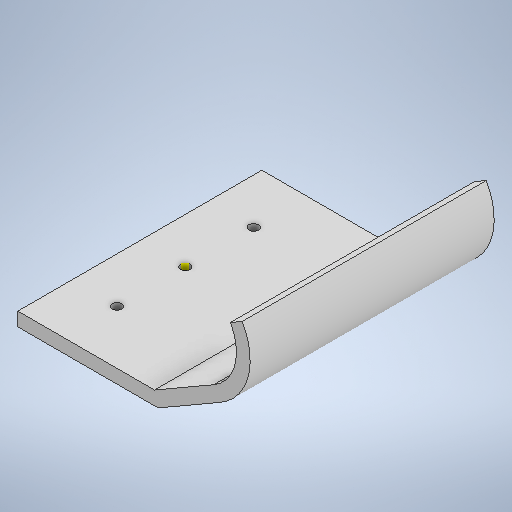
# Autodesk Inventor part: gripper_frame
Saved by Autodesk Inventor 2025.2 (Build 292293000, 293)
## iProperties
Created: 2025-08-01
Part Number: gripper_frame
Material: Generic
Document SubType Name: Modeling
Designer: LG
Density: 1 g/cm^3
Appearance: Default
Author: LG
Autodesk Inventor part; units mm, degrees
ref_plane "YZ Plane" through (0, 0, 0) normal (1, 0, 0) x (0, 1, 0)
ref_plane "XZ Plane" through (0, 0, 0) normal (0, 1, 0) x (-1, 0, 0)
ref_plane "XY Plane" through (0, 0, 0) normal (0, 0, 1) x (1, 0, 0)
sketch "Sketch1" plane through (0, 0, 0) normal (0, 1, 0) x (-1, 0, 0)
  line L0 (10, 26.78) -> (-20, 26.78)
  line L1 (-20, 26.78) -> (-20, -26.78)
  line L2 (-20, -26.78) -> (10, -26.78)
  line L3 (10, -26.78) -> (10, 26.78)
  point P0 (0, 0)
  dimension "d0" = 53.56
  dimension "d1" = 30
  dimension "d2" = 10
  dimension "d3" = 26.78
  constraints: 8 end point, 2 parallel, 1 horizontal, 1 perpendicular
  measures "d0" distance of L2.end L0.start
  measures "d1" distance of L1.end L2.end
  measures "d2" distance from line of point (0, 0) L3
  measures "d3" distance from line of L0 point (0, 0)
extrude "Extrusion1" add sketch "Sketch1" along normal blind 3
sketch "Sketch2" plane through (0, 3, 0) normal (0, 1, 0) x (1, 0, 0)
  circle A0 centre (-0.04, 0) radius 1.05
  line L0 (20, -26.78) -> (20, 26.78) projected
  circle A1 centre (-0.04, -15) radius 1.05
  circle A2 centre (-0.04, 15) radius 1.05
  point P0 (0, 0)
  point P1 (20, 0)
  dimension "d6" = 2.1
  dimension "d7" = 20.04
  dimension "d8" = 0
  dimension "d9" = 2.1
  dimension "d10" = 20.04
  dimension "d11" = 15
  dimension "d12" = 2.1
  dimension "d13" = 20.04
  dimension "d14" = 15
  constraints: 3 centre point, 1 midpoint
  measures "d6" diameter of A0
  measures "d7" distance of point (20, 0) A0.centre
  measures "d8" vertical distance of point (0, 0) A0.centre
  measures "d9" diameter of A1
  measures "d10" distance from line of L0 A1.centre
  measures "d11" vertical distance of point (0, 0) A1.centre
  measures "d12" diameter of A2
  measures "d13" distance from line of L0 A2.centre
  measures "d14" vertical distance of A2.centre point (0, 0)
extrude "Extrusion2" cut sketch "Sketch2" against normal blind 3
sketch "Sketch3" plane through (0, 3, 0) normal (0, 1, 0) x (1, 0, 0)
  point P0 (0, 0)
sketch "Sketch4" plane through (20, 0, 26.78) normal (1, 0, 0) x (0, 0, -1)
  line L0 (0, 3) -> (53.56, 3)
  line L1 (53.56, 3) -> (53.56, 0)
  line L2 (53.56, 0) -> (0, 0)
  line L3 (0, 0) -> (0, 3)
  line L4 (0, 3) -> (53.56, 3) projected
  line L5 (0, 0) -> (0, 3) projected
  point P0 (26.78, 0)
  dimension "d17" = 3
  dimension "d18" = 53.56
  dimension "d19" = 0
  dimension "d20" = 0
  constraints: 8 end point, 2 parallel, 1 horizontal, 1 perpendicular
  measures "d17" distance between parallel lines of L2 L0
  measures "d18" distance between parallel lines of L3 L1
  measures "d19" distance between parallel lines of L0 L4
  measures "d20" distance between parallel lines of L5 L3
revolve "Revolution2" add sketch "Sketch4" angle 30 about axis through (20, 3, 26.78) along (0, 0, 1)
sketch "Sketch6" plane through (20, 3, 26.78) normal (0.8660254, 0.5, 0) x (0, 0, -1)
  line L0 (0, 0) -> (53.56, 0)
  line L1 (53.56, 0) -> (53.56, -3)
  line L2 (53.56, -3) -> (0, -3)
  line L3 (0, -3) -> (0, 0)
  line L4 (0, 0) -> (53.56, 0) projected
  line L5 (0, 0) -> (0, -3) projected
  point P0 (26.78, 7.4019)
  dimension "d26" = 53.56
  dimension "d27" = 3
  dimension "d28" = 0
  dimension "d29" = 0
  constraints: 8 end point, 2 parallel, 1 horizontal, 1 perpendicular
  measures "d26" distance of L1.end L2.end
  measures "d27" distance of L2.end L0.start
  measures "d28" distance between parallel lines of L4 L0
  measures "d29" distance between parallel lines of L5 L3
extrude "Extrusion3" add sketch "Sketch6" along normal blind 15
sketch "Sketch7" plane through (32.9904, 10.5, 26.78) normal (0.8660254, 0.5, 0) x (0, 0, -1)
  line L0 (0, 0) -> (53.56, 0)
  line L1 (53.56, 0) -> (53.56, -3)
  line L2 (53.56, -3) -> (0, -3)
  line L3 (0, -3) -> (0, 0)
  line L4 (0, -3) -> (53.56, -3) projected
  line L5 (0, 0) -> (0, -3) projected
  point P0 (26.78, 7.4019)
  dimension "d32" = 53.56
  dimension "d33" = 3
  dimension "d34" = 0
  dimension "d35" = 0
  constraints: 8 end point, 2 parallel, 1 horizontal, 1 perpendicular
  measures "d32" distance of L0.start L0.end
  measures "d33" distance of L0.end L1.end
  measures "d34" distance between parallel lines of L4 L2
  measures "d35" distance between parallel lines of L5 L3
sketch "Sketch8" plane through (32.9904, 10.5, 26.78) normal (0.8660254, 0.5, 0) x (0, 0, -1)
  line L0 (-5.6464, 10) -> (58.6102, 10)
  line L1 (58.6102, 10) -> (58.6102, -7.2897)
  line L2 (58.6102, -7.2897) -> (-5.6464, -7.2897)
  line L3 (-5.6464, -7.2897) -> (-5.6464, 10)
  line L4 (53.56, 0) -> (0, 0) projected
  line L5 (53.56, -3) -> (53.56, 0) projected
  point P0 (26.78, 7.4019)
  dimension "d38" = 64.2566
  dimension "d39" = 17.2897
  dimension "d40" = 10
  dimension "d41" = 5.0502
  constraints: 8 end point, 2 parallel, 1 horizontal, 1 perpendicular
  measures "d38" distance of L1.end L2.end
  measures "d39" distance of L0.end L1.end
  measures "d40" distance between parallel lines of L4 L0
  measures "d41" distance between parallel lines of L5 L1
revolve "Revolution4" add sketch "Sketch7" angle 90 about axis through (27.9904, 19.1603, 32.4264) along (0, 0, 1)
body "Solid1"
